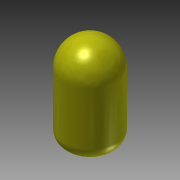
# Autodesk Inventor part: minion-body
Saved by Autodesk Inventor 2015 (Build 190159000, 159)
## iProperties
Created: 2014-12-10
Part Number: minion-body
Material: PAEK Plastic
Document SubType Name: Modeling
Designer: joe
Density: 1.32 g/cm^3
Appearance: Yellow
Author: joe
Autodesk Inventor part; units mm, degrees
ref_plane "YZ Plane" through (0, 0, 0) normal (1, 0, 0) x (0, 1, 0)
ref_plane "XZ Plane" through (0, 0, 0) normal (0, 1, 0) x (-1, 0, 0)
ref_plane "XY Plane" through (0, 0, 0) normal (0, 0, 1) x (1, 0, 0)
sketch "Sketch1" plane through (0, 0, 0) normal (0, 1, 0) x (-1, 0, 0)
  circle A0 centre (0, 0) radius 12.7
  point P0 (0, -12.7)
  dimension "d0" = 25.4
  constraints: 1 coincident, 1 vertical alignment, 2 other
extrude "Extrusion1" add sketch "Sketch1" along normal blind 44.45
fillet "Fillet1" radius 12.7 1 edges at (12.7, 44.45, 0)
fillet "Fillet2" radius 6.35 1 edges at (12.7, 0, 0)
body "Solid1"
